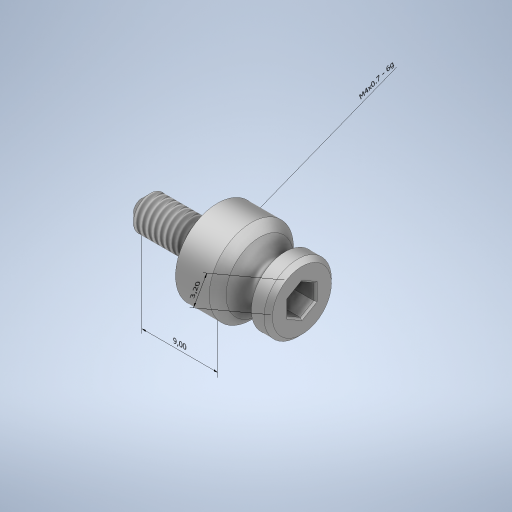
# Autodesk Inventor part: knob
Saved by Autodesk Inventor 2024 (Build 280153000, 153)
## iProperties
Created: 2023-09-10
Part Number: knob
Material: 铝 6061-AHC
Document SubType Name: Modeling
Designer: nicx5
Density: 2.7 g/cm^3
Appearance: 阳极电镀 - 浅灰色
Author: nicx5
Autodesk Inventor part; units mm, degrees
ref_plane "YZ Plane" through (0, 0, 0) normal (1, 0, 0) x (0, 1, 0)
ref_plane "XZ Plane" through (0, 0, 0) normal (0, 1, 0) x (-1, 0, 0)
sketch "草图1" plane through (0, 0, 0) normal (1, 0, 0) x (0, 1, 0)
  circle A0 centre (0, 0) radius 2
  circle A1 centre (0, 0) radius 5
  dimension "d0" = 4
  dimension "d1" = 10
  constraints: 2 centre point
  measures "d0" diameter of A0
  measures "d1" diameter of A1
extrude "拉伸1" add sketch "草图1" along normal blind 5 contours A0 | A1
extrude "拉伸2" add sketch "草图1" against normal blind 9 contours A0
chamfer "倒角1" distance 1 angle 45 1 edges at (-9, -2, 0)
thread "螺纹1" size "M4x0.7" class "6g" standard "ANSI Metric M Profile" length 9
ref_plane "工作平面2" through (8, 0, 0) normal (1, 0, 0) x (0, 0, -1)
ref_plane "工作平面1" through (6.5, 0, 0) normal (1, 0, 0) x (0, 0, -1)
sketch "草图3" plane through (8, 0, 0) normal (1, 0, 0) x (0, 0, -1)
  circle A0 centre (0, 0) radius 4
  dimension "d14" = 8
  constraints: 1 centre point
  measures "d14" diameter of A0
extrude "拉伸3" add sketch "草图3" along normal blind 2
chamfer "倒角3" distance 1 angle 45 1 edges at (5, -5, 0)
sketch "草图4" plane through (6.5, 0, 0) normal (1, 0, 0) x (0, 0, -1)
  circle A0 centre (0, 0) radius 2.5
  dimension "d29" = 5
  constraints: 1 centre point
  measures "d29" diameter of A0
loft "放样2" add profiles "草图4" section 1 edges at (5, -4, 0) section 3 edges at (8, 0, 4)
chamfer "倒角4" distance 0.5 angle 45 1 edges at (10, 0, 4)
sketch "草图6" plane through (10, 0, 0) normal (1, 0, 0) x (0, 0, -1)
  circle A0 centre (0, 0) radius 1.6
  line L0 (1.599, -0.9232) -> (0, -1.8464)
  line L1 (0, -1.8464) -> (-1.599, -0.9232)
  line L2 (-1.599, -0.9232) -> (-1.599, 0.9232)
  line L3 (-1.599, 0.9232) -> (0, 1.8464)
  line L4 (0, 1.8464) -> (1.599, 0.9232)
  line L5 (1.599, 0.9232) -> (1.599, -0.9232)
  dimension "d46" = 3.2
  constraints: 12 end point, 1 centre point, 13 other
  measures "d46" diameter of A0
extrude "拉伸5" cut sketch "草图6" against normal blind 4
chamfer "倒角6" distance 0.2 angle 45 6 edges at (10, 1.3848, -0.7995) (10, 1.3848, 0.7995) (10, 0, 1.599) (10, -1.3848, 0.7995) (10, -1.3848, -0.7995) (10, 0, -1.599)
chamfer "倒角7" distance 0.2 angle 45 6 edges at (6, 1.3848, 0.7995) (6, 1.3848, -0.7995) (6, 0, 1.599) (6, -1.3848, 0.7995) (6, -1.3848, -0.7995) (6, 0, -1.599)
